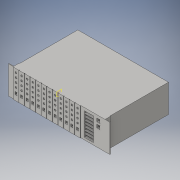
# Autodesk Inventor part: preamp
Saved by Autodesk Inventor 2016 (Build 200138000, 138)
## iProperties
Created: 2016-08-08
Part Number: preamp
Material: Generic
Document SubType Name: Modeling
Designer: Zuhra Abdurashidova
Density: 1 g/cm^3
Appearance: Default
Sheet Metal Rule: Default
Author: Zuhra Abdurashidova
Autodesk Inventor part; units mm, degrees
ref_plane "YZ Plane" through (0, 0, 0) normal (1, 0, 0) x (0, 1, 0)
ref_plane "XZ Plane" through (0, 0, 0) normal (0, 1, 0) x (-1, 0, 0)
ref_plane "XY Plane" through (0, 0, 0) normal (0, 0, 1) x (1, 0, 0)
sketch "Sketch2" plane through (0, 0, 0) normal (0, 1, 0) x (-1, 0, 0)
  line L0 (215.9, 152.4) -> (-215.9, 152.4)
  line L1 (-215.9, 152.4) -> (-215.9, -152.4)
  line L2 (-215.9, -152.4) -> (215.9, -152.4)
  line L3 (215.9, -152.4) -> (215.9, 152.4)
  line L4 (215.9, 152.4) -> (-215.9, -152.4) construction
  line L5 (-215.9, 152.4) -> (215.9, -152.4) construction
  point P0 (0, 0)
  point P1 (0, -152.4)
  dimension "d6" = 431.8
  dimension "d7" = 304.8
  constraints: 12 end point, 3 midpoint, 2 parallel, 1 horizontal, 1 perpendicular
  measures "d6" distance of L1.end L2.end
  measures "d7" distance of L0.end L1.end
extrude "preamp body" add sketch "Sketch2" along normal blind 133.35
ref_plane "Work Plane3" through (0, 133.35, 152.4) normal (1, 0, 0) x (0, 1, 0)
sketch "Sketch4" plane through (0, 133.35, 0) normal (0, 1, 0) x (1, 0, 0)
  line L0 (-215.9, -152.4) -> (215.9, -152.4) projected
  line L1 (215.9, -127) -> (215.9, -152.4)
  line L2 (215.9, -152.4) -> (241.3, -152.4)
  line L3 (241.3, -149.7584) -> (218.5416, -149.7584)
  line L4 (218.5416, -149.7584) -> (218.5416, -127)
  line L5 (215.9, -127) -> (218.5416, -127)
  line L6 (215.9, -152.4) -> (215.9, 152.4) projected
  line L7 (241.3, -152.4) -> (241.3, -149.7584)
  point P0 (0, 0)
  dimension "d13" = 25.4
  dimension "d14" = 25.4
  dimension "d15" = 2.6416
  constraints: 12 end point, 4 perpendicular, 1 vertical, 1 other
  measures "d13" distance of L0.end L2.end
  measures "d14" distance of L1.start L0.end
  measures "d15" distance between parallel lines of L3 L2
extrude "bracket" add sketch "Sketch4" against normal blind 133.35
mirror "Mirror1" about plane through (0, 133.35, 152.4) normal (1, 0, 0) of "bracket"
sketch "Sketch5" plane through (241.3, 0, 152.4) normal (0, 0, 1) x (1, 0, 0)
  line L0 (-457.2, 0) -> (-457.2, 133.35) projected
  line L1 (-457.2, 133.35) -> (-431.8, 133.35)
  line L2 (-431.8, 133.35) -> (-431.8, 0)
  line L3 (-431.8, 0) -> (-457.2, 0)
  line L4 (-457.2, 0) -> (-457.2, 133.35)
  point P0 (-241.3, 0)
  dimension "d18" = 25.4
  constraints: 8 end point, 2 parallel, 1 horizontal, 1 perpendicular
  measures "d18" distance of L0.end L1.end
extrude "eurocard" add sketch "Sketch5" along normal blind 2.54
sketch "Sketch8" plane through (241.3, 0, 154.94) normal (0, 0, 1) x (1, 0, 0)
  line L0 (-439.881, 116.6498) -> (-442.1905, 112.6497)
  line L1 (-442.1905, 112.6497) -> (-446.8095, 112.6497)
  line L2 (-446.8095, 112.6497) -> (-449.119, 116.6498)
  line L3 (-449.119, 116.6498) -> (-446.8095, 120.65)
  line L4 (-446.8095, 120.65) -> (-442.1905, 120.65)
  line L5 (-442.1905, 120.65) -> (-439.881, 116.6498)
  line L6 (-431.8, 133.35) -> (-457.2, 133.35) projected
  line L7 (-457.2, 133.35) -> (-457.2, 0) projected
  line L8 (-431.8, 0) -> (-431.8, 133.35) projected
  point P0 (-241.3, 0)
  point P1 (-444.5, 116.6498)
  dimension "d40" = 9.238
  dimension "d42" = 12.7
  dimension "d44" = 12.7
  dimension "d45" = 90
  constraints: 12 end point, 13 other
  measures "d40" distance of L0.start L2.end
  measures "d42" distance from line of L6 L4.end
  measures "d44" distance from line of point (-444.5, 116.65) L7
  measures "d45" angle of L8 L4
sketch "Sketch9" plane through (241.3, 0, 152.4) normal (0, 0, 1) x (1, 0, 0)
  line L0 (-121.3857, 120.3412) -> (-77.226, 120.3412)
  line L1 (-77.226, 120.3412) -> (-77.226, 108.3864)
  line L2 (-77.226, 108.3864) -> (-121.3857, 108.3864)
  line L3 (-121.3857, 108.3864) -> (-121.3857, 120.3412)
  point P0 (-241.3, 0)
  constraints: 8 end point, 2 parallel, 1 horizontal, 1 perpendicular
extrude "db25" cut sketch "Sketch9" against normal blind 25.4
sketch "Sketch10" plane through (241.3, 0, 152.4) normal (0, 0, 1) x (1, 0, 0)
  line L0 (-61.0775, 120.1521) -> (-46.7953, 120.1521)
  line L1 (-46.7953, 120.1521) -> (-46.7953, 104.7948)
  line L2 (-46.7953, 104.7948) -> (-61.0775, 104.7948)
  line L3 (-61.0775, 104.7948) -> (-61.0775, 120.1521)
  point P0 (-241.3, 0)
  constraints: 8 end point, 2 parallel, 1 horizontal, 1 perpendicular
extrude "Power" cut sketch "Sketch10" against normal blind 25.4
pattern_linear "Rectangular Pattern4" count 2 spacing 25.4 along (0, -1, 0) of "Power"
extrude "sma" cut sketch "Sketch8" against normal blind 2.54
pattern_linear "Rectangular Pattern5" count 4 spacing 20.32 along (0, -1, 0) of "sma"
sketch "Sketch11" plane through (241.3, 0, 154.94) normal (0, 0, 1) x (1, 0, 0)
  line L0 (-449.2072, 24.9355) -> (-439.7928, 24.9355)
  line L1 (-439.7928, 24.9355) -> (-439.7928, 37.2656)
  line L2 (-439.7928, 37.2656) -> (-449.2072, 37.2656)
  line L3 (-449.2072, 37.2656) -> (-449.2072, 24.9355)
  line L4 (-444.5, 12.7) -> (-444.5, 120.65) projected
  line L5 (-449.2072, 24.9355) -> (-439.7928, 37.2656) construction
  line L6 (-439.7928, 24.9355) -> (-449.2072, 37.2656) construction
  point P0 (-241.3, 0)
  point P1 (-444.5, 31.1005)
  constraints: 12 end point, 2 midpoint, 2 parallel, 1 horizontal, 1 perpendicular, 1 point on line
extrude "rj45" cut sketch "Sketch11" against normal blind 25.4
pattern_linear "Rectangular Pattern6" count 12 spacing 26.67 along (1, 0, 0) of "eurocard", "sma", "Rectangular Pattern5", "rj45"
pattern_linear "Rectangular Pattern7" count 8 spacing 13.97 along (0, -1, 0) of "db25"
equation "\"BendRadius\" = Thickness"
equation "\"BendReliefWidth\" = Thickness"
equation "\"BendReliefDepth\" = 0.5 * Thickness"
equation "\"CornerReliefSize\" = 4 * Thickness"
equation "\"MinimumRemnant\" = 2 * Thickness"
equation "\"TransitionRadius\" = BendRadius"
equation "\"JacobiRadiusSize\" = Thickness"
equation "\"GapSize\" = Thickness"
equation "\"Thickness\" = 3.048"
body "Solid3"
